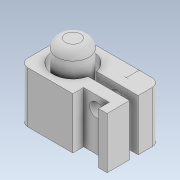
# Autodesk Inventor part: BOUCHON
Saved by Autodesk Inventor 2020 (Build 240168000, 168)
## iProperties
Created: 2020-07-01
Part Number: BOUCHON
Material: Generic
Document SubType Name: Modeling
Designer: Admin
Density: 1 g/cm^3
Appearance: Default
Author: Admin
Autodesk Inventor part; units mm, degrees
ref_plane "YZ Plane" through (0, 0, 0) normal (1, 0, 0) x (0, 1, 0)
ref_plane "XZ Plane" through (0, 0, 0) normal (0, 1, 0) x (-1, 0, 0)
ref_plane "XY Plane" through (0, 0, 0) normal (0, 0, 1) x (1, 0, 0)
sketch "Sketch1" plane through (0, 0, 0) normal (0, 1, 0) x (-1, 0, 0)
  circle A0 centre (0, 0) radius 3.75
  dimension "d0" = 7.5
  constraints: 1 centre point, 1 coincident
  measures "d0" diameter of A0
extrude "Extrusion1" add sketch "Sketch1" along normal blind 15
fillet "Fillet1" radius 2 1 edges at (3.75, 15, 0)
sketch "Sketch2" plane through (0, 0, 0) normal (0, -1, 0) x (1, 0, 0)
  line L0 (14.25, 6.25) -> (-6.25, 6.25)
  line L1 (-6.25, 6.25) -> (-6.25, -6.25)
  line L2 (-6.25, -6.25) -> (14.25, -6.25)
  line L3 (14.25, -6.25) -> (14.25, 6.25)
  point P0 (0, 0)
  dimension "d4" = 12.5
  dimension "d5" = 20.5
  dimension "d6" = 6.25
  dimension "d7" = 6.25
  constraints: 8 end point, 2 parallel, 1 horizontal, 1 perpendicular
  measures "d4" distance of L0.end L1.end
  measures "d5" distance of L0.start L0.end
  measures "d6" distance from line of L1 point (0, 0)
  measures "d7" distance from line of L2 point (0, 0)
extrude "Extrusion2" add sketch "Sketch2" along normal blind 2
sketch "Sketch3" plane through (0, 0, 0) normal (0, 1, 0) x (1, 0, 0)
  line L0 (14.25, -6.25) -> (-6.25, -6.25) projected
  line L1 (-6.25, 6.25) -> (14.25, 6.25) projected
  line L2 (-6.25, -6.25) -> (14.25, -6.25)
  line L3 (14.25, -6.25) -> (14.25, 6.25)
  line L4 (14.25, 6.25) -> (-6.25, 6.25)
  line L5 (-6.25, 6.25) -> (-6.25, -6.25)
  circle A0 centre (0, 0) radius 4.65
  point P0 (-6.25, 6.25)
  dimension "d10" = 9.3
  constraints: 8 end point, 2 parallel, 1 centre point, 1 coincident, 1 horizontal, 1 perpendicular
  measures "d10" diameter of A0
extrude "Extrusion3" add sketch "Sketch3" along normal blind 10
sketch "Sketch4" plane through (14.25, -2, 6.25) normal (1, 0, 0) x (0, 0, -1)
  line L0 (5.25, 0) -> (7.25, 0)
  line L1 (7.25, 0) -> (7.25, 12)
  line L2 (7.25, 12) -> (5.25, 12)
  line L3 (5.25, 12) -> (5.25, 0)
  line L4 (12.5, 0) -> (0, 0) projected
  line L5 (0, 12) -> (12.5, 12) projected
  line L6 (0, 12) -> (0, 0) projected
  point P0 (6.25, 2)
  dimension "d14" = 2
  dimension "d15" = 5.25
  constraints: 8 end point, 2 parallel, 2 point on line, 1 horizontal, 1 perpendicular
  measures "d14" distance of L1.end L2.end
  measures "d15" distance between parallel lines of L6 L3
extrude "Extrusion4" cut sketch "Sketch4" against normal blind 9.71 contours L3 L2 L1 L0
sketch "Sketch6" plane through (0, 10, 0) normal (0, 1, 0) x (1, 0, 0)
  line L0 (6.25, -6.25) -> (12.25, -6.25)
  line L1 (12.25, -6.25) -> (12.25, -3.75)
  line L2 (12.25, -3.75) -> (6.25, -3.75)
  line L3 (6.25, -3.75) -> (6.25, -6.25)
  line L4 (14.25, -6.25) -> (14.25, -1) projected
  line L5 (-6.25, -6.25) -> (14.25, -6.25) projected
  point P0 (0, 0)
  dimension "d18" = 6
  dimension "d19" = 2.5
  dimension "d20" = 2
  constraints: 8 end point, 2 parallel, 1 horizontal, 1 perpendicular, 1 point on line
  measures "d18" distance of L0.start L0.end
  measures "d19" distance of L2.end L0.start
  measures "d20" distance between parallel lines of L4 L1
extrude "Extrusion5" cut sketch "Sketch6" against normal through all
sketch "Sketch7" plane through (14.25, -2, -6.25) normal (0, 0, -1) x (-1, 0, 0)
  circle A0 centre (5, 9) radius 1.6
  line L0 (0, 12) -> (20.5, 12) projected
  line L1 (0, 12) -> (0, 0) projected
  point P0 (14.25, 2)
  dimension "d23" = 3.2
  dimension "d24" = 3
  dimension "d25" = 5
  constraints: 1 centre point
  measures "d23" diameter of A0
  measures "d24" distance from line of L0 A0.centre
  measures "d25" distance from line of L1 A0.centre
extrude "Extrusion6" cut sketch "Sketch7" against normal through all
sketch "Sketch8" plane through (14.25, -2, -6.25) normal (0, 0, -1) x (-1, 0, 0)
  circle A0 centre (5, 9) radius 3
  line L0 (0, 12) -> (20.5, 12) projected
  line L1 (0, 12) -> (0, 0) projected
  point P0 (14.25, 2)
  dimension "d28" = 6
  dimension "d29" = 3
  dimension "d30" = 5
  constraints: 1 centre point
  measures "d28" diameter of A0
  measures "d29" distance from line of L0 A0.centre
  measures "d30" distance from line of A0.centre L1
extrude "Extrusion7" cut sketch "Sketch8" against normal blind 3
fillet "Fillet2" radius 2 3 edges at (-6.25, 4, -6.25) (14.25, 4, -6.25) (-6.25, 4, 6.25)
equation "\"d7\" = d6"
body "Solid1"
